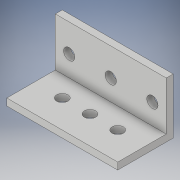
# Autodesk Inventor part: ball gripper to hatch attachment
Saved by Autodesk Inventor 2018 (Build 220112000, 112)
## iProperties
Created: 2019-03-04
Part Number: ball gripper to hatch attachment
Material: Generic
Document SubType Name: Modeling
Designer: Tiberus
Density: 1 g/cm^3
Appearance: Default
Author: Tiberus
Autodesk Inventor part; units mm, degrees
ref_plane "YZ Plane" through (0, 0, 0) normal (1, 0, 0) x (0, 1, 0)
ref_plane "XZ Plane" through (0, 0, 0) normal (0, 1, 0) x (-1, 0, 0)
ref_plane "XY Plane" through (0, 0, 0) normal (0, 0, 1) x (1, 0, 0)
sketch "Sketch1" plane through (0, 0, 0) normal (1, 0, 0) x (0, 1, 0)
  line L0 (0, 0) -> (3.175, 0)
  line L1 (3.175, 0) -> (3.175, -22.225)
  line L2 (3.175, -25.4) -> (0, -25.4)
  line L3 (0, -25.4) -> (0, 0)
  line L4 (3.175, -25.4) -> (25.4, -25.4)
  line L5 (25.4, -25.4) -> (25.4, -22.225)
  line L6 (25.4, -22.225) -> (3.175, -22.225)
  line L7 (3.175, -22.225) -> (3.175, -25.4)
  dimension "d0" = 3.175
  dimension "d1" = 25.4
  dimension "d2" = 22.225
  dimension "d3" = 3.175
  constraints: 16 end point, 4 parallel, 2 horizontal, 2 perpendicular
  measures "d0" distance of L2.start L2.end
  measures "d1" distance of L0.end L2.start
  measures "d2" distance of L1.end L5.end
  measures "d3" distance of L5.end L4.end
extrude "Extrusion1" add sketch "Sketch1" along normal blind 50.8
sketch "Sketch2" plane through (0, 3.175, 0) normal (0, 1, 0) x (1, 0, 0)
  line L0 (0, 0) -> (0, 25.4) construction
  line L1 (0, 12.7) -> (12.7, 12.7) construction
  line L2 (12.7, 12.7) -> (12.7, 0) construction
  line L3 (0, 0) -> (50.8, 0) construction
  line L4 (25.4, 12.7) -> (38.1, 12.7) construction
  circle A0 centre (12.7, 12.7) radius 2.5797
  circle A1 centre (25.4, 12.7) radius 2.5797
  circle A2 centre (38.1, 12.7) radius 2.5797
  dimension "d6" = 12.7
  dimension "d7" = 12.7
  dimension "d8" = 5.1594
  dimension "d9" = 5.1594
  dimension "d10" = 5.1594
  constraints: 6 end point, 3 centre point, 3 coincident, 3 point on line, 1 horizontal, 1 midpoint, 1 perpendicular
  measures "d6" distance of L1.start L1.end
  measures "d7" distance of L4.start L4.end
  measures "d8" diameter of A0
  measures "d9" diameter of A1
  measures "d10" diameter of A2
extrude "Extrusion2" cut sketch "Sketch2" against normal blind 50.8
sketch "Sketch3" plane through (0, 3.175, -22.225) normal (0, 0, 1) x (1, 0, 0)
  line L0 (0, 22.225) -> (0, 0) construction
  line L1 (50.8, 22.225) -> (50.8, 0) construction
  line L2 (0, 22.225) -> (50.8, 22.225) construction
  line L3 (25.4, 22.225) -> (25.4, 9.525) construction
  line L4 (25.4, 9.525) -> (44.45, 9.525) construction
  line L5 (25.4, 9.525) -> (6.35, 9.525) construction
  circle A0 centre (25.4, 9.525) radius 2.5797
  circle A1 centre (44.45, 9.525) radius 2.5797
  circle A2 centre (6.35, 9.525) radius 2.5797
  point P0 (0, -3.175)
  dimension "d22" = 12.7
  dimension "d23" = 19.05
  dimension "d24" = 19.05
  dimension "d25" = 5.1594
  dimension "d26" = 5.1594
  dimension "d27" = 5.1594
  constraints: 6 end point, 3 centre point, 3 coincident, 1 horizontal, 1 midpoint, 1 perpendicular, 1 vertical
  measures "d22" distance of L3.start L3.end
  measures "d23" distance of L3.end L4.end
  measures "d24" distance of L3.end L5.end
  measures "d25" diameter of A0
  measures "d26" diameter of A1
  measures "d27" diameter of A2
extrude "Extrusion3" cut sketch "Sketch3" against normal blind 50.8
body "Solid1"
